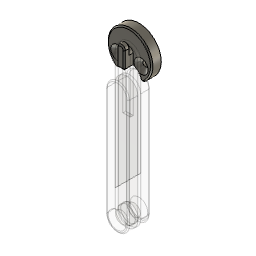
model (Autodesk Fusion 360 design; units mm, degrees)
Autodesk Fusion 360 part; units mm, degrees
sketch "Sketch1" plane through (0, 0, 0) normal (0, 1, 0) x (1, 0, 0)
  line L0 (0, 0) -> (0, -117.3)
  arc A0 (0, -117.3) -> (19.2, -117.3) centre (9.6, -117.3) ccw
  line L1 (19.2, -117.3) -> (19.2, 0)
  arc A1 (19.2, 0) -> (0, 0) centre (9.6, 0) ccw
  arc A2 (0, -92.8) -> (19.2, -92.8) centre (9.6, -92.8) ccw
  line L2 (6.425, -101.8598) -> (6.425, -119.925)
  arc A3 (6.425, -119.925) -> (12.775, -119.925) centre (9.6, -119.925) ccw
  line L3 (12.775, -119.925) -> (12.775, -101.8598)
  line L4 (9.6, -117.3) -> (9.6, -119.925) construction
  line L5 (0, -14.9) -> (19.2, -34.1)
  circle A4 centre (9.6, 0) radius 7.5
  line L6 (6.425, -101.8598) -> (6.425, -73.65)
  line L7 (12.775, -73.65) -> (12.775, -101.8598)
  line L8 (6.425, -73.65) -> (12.775, -73.65)
  point P0 (9.6, -102.4)
  point P1 (9.6, 9.6)
  point P2 (9.6, -126.9)
  point P3 (9.6, -123.1)
  dimension "d1" = 19.2
  dimension "d2" = 112
  dimension "d3" = 24.5
  dimension "d4" = 3.8
  dimension "d5" = 6.35
  dimension "d6" = 45
  dimension "d7" = 15
  dimension "d8" = 112
  dimension "d10" = 49.45
  constraint coincident L0.start A1.end
  constraint vertical L0
  constraint tangent L0 A0
  constraint tangent A0 L1
  constraint tangent L1 A1
  constraint tangent L0 A1
  constraint coincident L1 A2.end
  constraint coincident L0 A2.start
  constraint tangent L0 A2
  constraint tangent L1 A2
  constraint coincident A2 L2.start
  constraint tangent L2 A3
  constraint coincident A2 L3.end
  constraint tangent A3 L3
  constraint vertical L2
  constraint vertical L3
  constraint coincident A0.centre L4.start
  constraint coincident A3.centre L4.end
  constraint vertical L4
  constraint midpoint A2 P0
  constraint midpoint A1 P1
  constraint midpoint A0 P2
  constraint midpoint A3 P3
  constraint coincident L0 L5.start
  constraint coincident L1 L5.end
  constraint concentric A1 A4
  constraint vertical L6
  constraint vertical L7
  constraint vertical L1
  constraint horizontal L8
  measures "d1" distance of L0.start L1.end
  measures "d2" distance of P0 P1
  measures "d3" distance of P0 P2
  measures "d4" distance of P2 P3
  measures "d5" distance of L2.end A3.end
  measures "d6" angle of L0 L5
  measures "d7" diameter of A4
  measures "d8" vertical distance of P2 L5.start
  measures "d10" vertical distance of P3 L7.start
extrude "Extrude1" add sketch "Sketch1" along normal mid plane 2.45 contours L0 L1 A2 L5 L6 L7 L8 | L0 A0 L1 A2 L2 A3 L3 makes body 1
extrude "Extrude2" add sketch "Sketch1" against normal blind 8.125 from surface at -1.225 separate body contours L0 L1 A1 L5 | L0 L1 A2 L5 L6 L7 L8 | A2 L6 L7 L8 makes body 2
extrude "Extrude3" add sketch "Sketch1" along normal mid plane 15 separate body contours A4 makes body 3
fillet "Fillet1" radius 7.5 2 edges at (2.6075, -7.5, -2.7121) (2.6075, 7.5, 2.7121) on bodies 3
draft "Draft1" angle 30 neutral plane through (0, -9.35, 0) pull (0, -1, 0) 1 faces at (17.0627, -3.9333, 0.7468) on bodies 2
combine "Combine1" operation cut target body 2 tool bodies 3 keep tools
chamfer "Chamfer1" distance 1 angle 45 4 edges at (9.6, -9.35, 102.4) (0, -9.35, 46.4) (9.6, -9.35, -9.6) (19.2, -9.35, 46.4) on bodies 2
ref_plane "WorkPlane1" through (9.6, 0, 70.9) normal (0, -1, 0) x (-1, 0, 0)
mirror "Mirror1" about plane through (9.6, 0, 70.9) normal (0, -1, 0) of bodies 2 makes body 4
sketch "Sketch1 (2)" plane through (0, 9.35, 0) normal (0, 1, 0) x (-1, 0, 0) in component "mount"
  circle A0 centre (-9.6, 0) radius 7.5
  arc A1 (-1, 92.8) -> (-18.2, 92.8) centre (-9.6, 92.8) ccw
  line L0 (-18.2, 92.8) -> (-18.2, 0)
  arc A2 (-18.2, 0) -> (-1, 0) centre (-9.6, 0) ccw
  line L1 (-1, 0) -> (-1, 92.8)
  arc A3 (0, 92.8) -> (-19.2, 92.8) centre (-9.6, 92.8) ccw
  arc A4 (-19.2, 0) -> (0, 0) centre (-9.6, 0) ccw
  line L2 (-19.2, 0) -> (-19.2, 92.8)
  line L3 (0, 92.8) -> (0, 0)
  line L4 (-6.425, 119.925) -> (-6.425, 73.65)
  line L5 (-6.425, 73.65) -> (-12.775, 73.65)
  line L6 (-12.775, 73.65) -> (-12.775, 119.925)
  arc A5 (-6.425, 119.925) -> (-12.775, 119.925) centre (-9.6, 119.925) ccw
  arc A6 (0, 117.3) -> (-19.2, 117.3) centre (-9.6, 117.3) ccw
  line L7 (-19.2, 117.3) -> (-19.2, 34.1)
  line L8 (-19.2, 34.1) -> (0, 14.9)
  line L9 (0, 14.9) -> (0, 117.3)
  line L10 (-12.775, 119.925) -> (-12.775, 124.925)
  arc A7 (-6.425, 124.925) -> (-12.775, 124.925) centre (-9.6, 124.925) ccw
  line L11 (-6.425, 124.925) -> (-6.425, 119.925)
  arc A8 (-6.425, 107.0598) -> (-12.775, 107.0598) centre (-9.6, 98) ccw
  line L12 (-9.6, 98) -> (-9.6, 92.8) construction
  circle A9 centre (0.4, 113.4924) radius 2.25
  circle A10 centre (0.4, 113.4924) radius 6 construction
  line L13 (-6.425, 107.0598) -> (0.4, 113.4924) construction
  line L14 (-6.425, 119.925) -> (0.4, 113.4924) construction
  circle A11 centre (-19.6, 113.4924) radius 2.25
  circle A12 centre (-19.6, 113.4924) radius 6 construction
  circle A13 centre (-9.6, 117.3) radius 19
  arc A14 (0, 100.9037) -> (-19.2, 100.9037) centre (-9.6, 100.9037) ccw
  arc A15 (0, 92.8) -> (-19.2, 92.8) centre (-9.6, 92.8) ccw
  point P0 (-12.775, 101.8598)
  dimension "d25" = 5
  dimension "d26" = 5.2
  dimension "d27" = 12
  dimension "d28" = 4.5
  dimension "d29" = 20
  dimension "d30" = 38
  constraint coincident L6.end A5.end
  constraint tangent L10 A7
  constraint coincident L4.start A5.start
  constraint vertical L10
  constraint vertical L11
  constraint tangent A7 L11
  constraint coincident L4 A8.start
  constraint coincident L6 A8.end
  constraint equal A3 A8
  constraint coincident A8.centre L12.start
  constraint coincident A1.centre A3.centre
  constraint vertical L12
  constraint coincident A3 P0
  constraint coincident L6 P0
  constraint concentric A9 A10
  constraint coincident A9.centre A10.centre
  constraint equal L13 L14
  constraint symmetric L12 A9 A11
  constraint symmetric L12 A10 A12
  constraint concentric A6 A13
  constraint coincident L7 A14.end
  constraint coincident A13 A14.end
  constraint coincident A13 A14.start
  constraint coincident L9 A14.start
  constraint equal A14 A15
  measures "d25" distance of A5.centre A7.centre
  measures "d26" distance of A8.end P0
  measures "d27" diameter of A10
  measures "d28" diameter of A9
  measures "d29" distance of A9.centre A11.centre
  measures "d30" diameter of A13
extrude "Extrude1'" add sketch "Sketch1 (2)" against normal up to surface (8.125 mm away) separate body contours L4 A6 L9 A7 L11 A9 A14 | A6 L7 L9 A7 A9 A11 A13 | L4 L6 A5 A14 | L6 A6 L7 L10 A7 A11 A14 | A5 A6 L10 A7 L11 | A6 A7 makes body 5 in component "mount"
extrude "Extrude2'" add sketch "Sketch1 (2)" against normal up to surface (2.65 mm away) from surface at -8.125 contours L4 L6 A5 A14 bodies 5 in component "mount"
extrude "Extrude3'" add sketch "Sketch1 (2)" against normal blind 5 from surface at -10.775 contours L4 L6 A5 A14 | A5 A6 L10 A7 L11 | A6 A7 bodies 5 in component "mount"
chamfer "Chamfer1'" distance 3.75 angle 45 2 edges at (1.6977, 1.225, 112.6787) (21.6977, 1.225, 112.6787) on bodies 5 in component "mount"
fillet "Fillet1'" radius 1 2 edges at (6.425, -2.6, 109.9634) (12.775, -2.6, 109.9634) on bodies 5 in component "mount"
fillet "Fillet1'" radius 2 2 edges at (0, 5.2875, 100.9037) (19.2, 5.2875, 100.9037) on bodies 5 in component "mount"
chamfer "Chamfer2" distance 1 angle 45 14 edges at (9.6, 1.225, 136.3) (20.1134, 1.225, 102.4692) (16.0447, 1.225, 108.0188) (3.1553, 1.225, 108.0188) (-0.9134, 1.225, 102.4692) (6.425, -6.425, 118.1016) (6.7946, -6.425, 110.5018) (9.6, -6.425, 110.5037) (12.4054, -6.425, 110.5018) (12.775, -6.425, 118.1016) (9.6, -6.425, 128.1) (9.6, -1.425, 128.1) (6.425, -1.425, 122.425) (12.775, -1.425, 122.425) on bodies 5 in component "mount"
component "mount" placed x (1, 0, 0) y (0, 1, 0) z (0, 0, 1) at (0, 0, 0)
equation "d5 = 1/4\""
equation "d8 = d2"
equation "d11 = 2.45 mm"
equation "d14 = -( 18.7 mm - d11 ) / 2"
equation "d26 = d25 + 0.2 mm"
